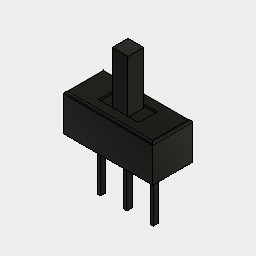
Enclosure Case for Circuit Playground (Autodesk Fusion 360 archive; units mm, degrees)
design "Slide Switch"
Autodesk Fusion 360 part; units mm, degrees
sketch "Sketch1" plane through (0, 0, 0) normal (0, 0, 1) x (1, 0, 0)
  line L0 (-4.25, -1.9) -> (4.25, -1.9)
  line L1 (4.25, -1.9) -> (4.25, 1.9)
  line L2 (4.25, 1.9) -> (-4.25, 1.9)
  line L3 (-4.25, 1.9) -> (-4.25, -1.9)
  line L4 (-4.25, -1.9) -> (4.25, 1.9) construction
  line L5 (4.25, -1.9) -> (-4.25, 1.9) construction
  dimension "d1" = 8.5
  dimension "d2" = 3.8
  measures "d1" distance of L1.end L2.end
  measures "d2" distance of L0.start L2.end
extrude "Extrude1" add sketch "Sketch1" along normal blind 3.5
sketch "Sketch2" plane through (0, 0, 3.5) normal (0, 0, 1) x (-1, 0, 0)
  line L0 (4.25, -1.9) -> (4.25, 1.9)
  line L1 (4.25, 1.9) -> (-4.25, 1.9)
  line L2 (-4.25, 1.9) -> (-4.25, -1.9)
  line L3 (-4.25, -1.9) -> (4.25, -1.9)
  line L4 (1.9, -0.9) -> (-1.9, -0.9)
  line L5 (-1.9, -0.9) -> (-1.9, 0.9)
  line L6 (-1.9, 0.9) -> (1.9, 0.9)
  line L7 (1.9, 0.9) -> (1.9, -0.9)
  line L8 (-1.9, 0.9) -> (1.9, -0.9) construction
  dimension "d5" = 3.8
  dimension "d6" = 1.8
  measures "d5" distance of L4.start L4.end
  measures "d6" distance of L4.end L5.end
extrude "Extrude2" cut sketch "Sketch2" against normal blind 0.2 contours L4 L5 L6 L7
sketch "Sketch3" plane through (0, 0, 3.3) normal (0, 0, 1) x (-1, 0, 0)
  line L0 (1.9, 0.9) -> (-1.9, 0.9)
  line L1 (-1.9, 0.9) -> (-1.9, -0.9)
  line L2 (-1.9, -0.9) -> (1.9, -0.9)
  line L3 (1.9, -0.9) -> (1.9, 0.9)
  line L4 (0.75, -0.75) -> (-0.75, -0.75)
  line L5 (-0.75, -0.75) -> (-0.75, 0.75)
  line L6 (-0.75, 0.75) -> (0.75, 0.75)
  line L7 (0.75, 0.75) -> (0.75, -0.75)
  line L8 (0.75, -0.75) -> (-0.75, 0.75) construction
  line L9 (-0.75, -0.75) -> (0.75, 0.75) construction
  dimension "d9" = 1.5
  dimension "d10" = 1.5
  measures "d9" distance of L5.end L6.end
  measures "d10" distance of L4.end L5.end
extrude "Extrude3" add sketch "Sketch3" along normal blind 5 contours L4 L5 L6 L7
sketch "Sketch4" plane through (0, 0, 0) normal (0, 0, -1) x (1, 0, 0)
  line L0 (-4.25, 1.9) -> (-4.25, -1.9)
  line L1 (-4.25, -1.9) -> (4.25, -1.9)
  line L2 (4.25, -1.9) -> (4.25, 1.9)
  line L3 (4.25, 1.9) -> (-4.25, 1.9)
  line L4 (-0.15, 0.25) -> (0.15, 0.25)
  line L5 (0.15, 0.25) -> (0.15, -0.25)
  line L6 (0.15, -0.25) -> (-0.15, -0.25)
  line L7 (-0.15, -0.25) -> (-0.15, 0.25)
  line L8 (0.15, -0.25) -> (-0.15, 0.25) construction
  line L9 (-2.35, -0.25) -> (-2.65, -0.25)
  line L10 (-2.65, -0.25) -> (-2.65, 0.25)
  line L11 (-2.65, 0.25) -> (-2.35, 0.25)
  line L12 (-2.35, 0.25) -> (-2.35, -0.25)
  line L13 (-2.35, -0.25) -> (-2.65, 0.25) construction
  line L14 (-2.65, -0.25) -> (-2.35, 0.25) construction
  line L15 (2.65, -0.25) -> (2.35, -0.25)
  line L16 (2.35, -0.25) -> (2.35, 0.25)
  line L17 (2.35, 0.25) -> (2.65, 0.25)
  line L18 (2.65, 0.25) -> (2.65, -0.25)
  line L19 (2.65, -0.25) -> (2.35, 0.25) construction
  line L20 (2.35, -0.25) -> (2.65, 0.25) construction
  point P0 (-2.5, 0)
  point P1 (2.5, 0)
  dimension "d16" = 0.3
  dimension "d17" = 0.5
  dimension "d18" = 0.3
  dimension "d19" = 0.5
  dimension "d20" = 2.5
  dimension "d21" = 0.5
  dimension "d22" = 0.3
  dimension "d23" = 2.5
  measures "d16" distance of L4.start L4.end
  measures "d17" distance of L4.end L5.end
  measures "d18" distance of L10.end L11.end
  measures "d19" distance of L9.start L11.end
  measures "d20" distance of origin P0
  measures "d21" distance of L15.end L16.end
  measures "d22" distance of L16.end L17.end
  measures "d23" distance of origin P1
extrude "Extrude4" add sketch "Sketch4" along normal blind 5 contours L4 L5 L6 L7 | L9 L10 L11 L12 | L15 L16 L17 L18
fillet "Fillet1" radius 0.2 4 edges at (0, -1.9, 3.5) (-4.25, 0, 3.5) (0, 1.9, 3.5) (4.25, 0, 3.5)
equation "d18 = d16"
equation "d19 = d17"
equation "d21 = d17"
equation "d22 = d16"
equation "d23 = d20"

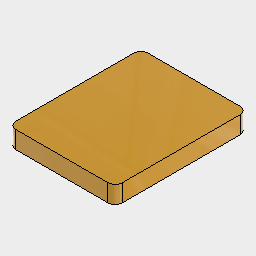
design "Battery"
Autodesk Fusion 360 part; units mm, degrees
sketch "Sketch1" plane through (0, 0, 0) normal (0, 0, 1) x (1, 0, 0)
  line L0 (-14.5, 18) -> (14.5, 18)
  line L1 (14.5, 18) -> (14.5, -18)
  line L2 (14.5, -18) -> (-14.5, -18)
  line L3 (-14.5, -18) -> (-14.5, 18)
  line L4 (-14.5, 18) -> (14.5, -18) construction
  line L5 (14.5, 18) -> (-14.5, -18) construction
  dimension "d1" = 36
  dimension "d2" = 29
  measures "d1" distance of L0.end L1.end
  measures "d2" distance of L1.end L2.end
extrude "Extrude1" add sketch "Sketch1" along normal blind 4.75
fillet "Fillet1" radius 2 4 edges at (-14.5, -18, 2.375) (-14.5, 18, 2.375) (14.5, 18, 2.375) (14.5, -18, 2.375)

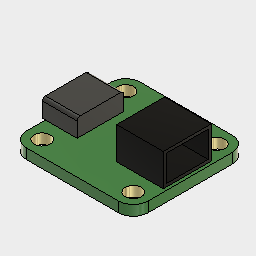
design "Battery Charger"
Autodesk Fusion 360 part; units mm, degrees
sketch "Sketch1" plane through (0, 0, 0) normal (0, 0, 1) x (1, 0, 0)
  line L0 (-10.16, 9.525) -> (10.16, 9.525)
  line L1 (10.16, 9.525) -> (10.16, -9.525)
  line L2 (10.16, -9.525) -> (-10.16, -9.525)
  line L3 (-10.16, -9.525) -> (-10.16, 9.525)
  line L4 (-10.16, 9.525) -> (10.16, -9.525) construction
  line L5 (10.16, 9.525) -> (-10.16, -9.525) construction
  circle A0 centre (-7.62, 6.985) radius 1.35
  circle A1 centre (7.62, 6.985) radius 1.35
  line L6 (0, 14.6922) -> (0, 11.826) construction
  line L7 (14.0724, 0) -> (17.9361, 0) construction
  circle A2 centre (-7.62, -6.985) radius 1.35
  circle A3 centre (7.62, -6.985) radius 1.35
  dimension "d1" = 20.32
  dimension "d2" = 19.05
  dimension "d3" = 2.7
  dimension "d4" = 15.24
  dimension "d5" = 13.97
  measures "d1" distance of L0.start L0.end
  measures "d2" distance of L0.end L1.end
  measures "d3" diameter of A0
  measures "d4" distance of A0.centre A1.centre
  measures "d5" distance of A1.centre A3.centre
extrude "Extrude1" add sketch "Sketch1" along normal blind 1.7
sketch "Sketch2" plane through (0, 0, 1.7) normal (0, 0, 1) x (-1, 0, 0)
  circle A0 centre (-7.62, -6.985) radius 1.35
  circle A1 centre (-7.62, 6.985) radius 1.35
  circle A2 centre (7.62, 6.985) radius 1.35
  circle A3 centre (7.62, -6.985) radius 1.35
  line L0 (10.16, 9.525) -> (-10.16, 9.525)
  line L1 (-10.16, 9.525) -> (-10.16, -9.525)
  line L2 (-10.16, -9.525) -> (10.16, -9.525)
  line L3 (10.16, -9.525) -> (10.16, 9.525)
  line L4 (-1.86, -4) -> (-9.66, -4)
  line L5 (-9.66, -4) -> (-9.66, 4)
  line L6 (-9.66, 4) -> (-1.86, 4)
  line L7 (-1.86, 4) -> (-1.86, -4)
  line L8 (-9.66, 4) -> (-1.86, -4) construction
  line L9 (4.86, 3.9) -> (10.66, 3.9)
  line L10 (10.66, 3.9) -> (10.66, -3.9)
  line L11 (10.66, -3.9) -> (4.86, -3.9)
  line L12 (4.86, -3.9) -> (4.86, 3.9)
  line L13 (4.86, 3.9) -> (10.66, -3.9) construction
  line L14 (10.66, 3.9) -> (4.86, -3.9) construction
  point P0 (-5.76, 0)
  point P1 (7.76, 0)
  dimension "d8" = 8
  dimension "d9" = 7.8
  dimension "d10" = 0.5
  dimension "d11" = 5.8
  dimension "d12" = 7.8
  dimension "d14" = 0.5
  measures "d8" distance of L4.end L5.end
  measures "d9" distance of L4.start L4.end
  measures "d10" distance of L1 L5
  measures "d11" distance of L10.end L11.end
  measures "d12" distance of L9.start L11.end
  measures "d14" distance of L3 L10
extrude "Extrude2" add sketch "Sketch2" along normal blind 5.4 contours L4 L5 L6 L7
extrude "Extrude3" add sketch "Sketch2" along normal blind 3 contours L3 L9 L10 L11 | L3 L9 L11 L12
sketch "Sketch3" plane through (9.66, 0, 0) normal (1, 0, 0) x (0, 1, 0)
  line L0 (-4, 1.7) -> (4, 1.7)
  line L1 (4, 1.7) -> (4, 7.1)
  line L2 (4, 7.1) -> (-4, 7.1)
  line L3 (-4, 7.1) -> (-4, 1.7)
  line L4 (-3.5, 2.2) -> (3.5, 2.2)
  line L5 (3.5, 2.2) -> (3.5, 6.6)
  line L6 (3.5, 6.6) -> (-3.5, 6.6)
  line L7 (-3.5, 6.6) -> (-3.5, 2.2)
  dimension "d19" = 0.5
extrude "Extrude4" cut sketch "Sketch3" against normal blind 5 contours L4 L5 L6 L7
sketch "Sketch4" plane through (-10.66, 0, 0) normal (-1, 0, 0) x (0, -1, 0)
  line L0 (-3.9, 1.7) -> (3.9, 1.7)
  line L1 (3.9, 1.7) -> (3.9, 4.7)
  line L2 (3.9, 4.7) -> (-3.9, 4.7)
  line L3 (-3.9, 4.7) -> (-3.9, 1.7)
  line L4 (-3.4, 2.2) -> (3.4, 2.2)
  line L5 (3.4, 2.2) -> (3.4, 4.2)
  line L6 (3.4, 4.2) -> (-3.4, 4.2)
  line L7 (-3.4, 4.2) -> (-3.4, 2.2)
  dimension "d22" = 0.5
extrude "Extrude5" cut sketch "Sketch4" against normal blind 4 contours L4 L5 L6 L7
fillet "Fillet1" radius 2.5 4 edges at (10.16, -9.525, 0.85) (-10.16, -9.525, 0.85) (-10.16, 9.525, 0.85) (10.16, 9.525, 0.85)
fillet "Fillet2" radius 0.5 4 edges at (-7.76, -3.9, 4.7) (-7.76, 3.9, 4.7) (-8.66, 3.4, 4.2) (-8.66, -3.4, 4.2)
